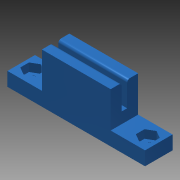
# Autodesk Inventor part: GT2 grip
Saved by Autodesk Inventor 2013 SP2 (Build 170200200, 200)
## iProperties
Created: 2017-01-29
Part Number: GT2 grip
Material: Generic
Document SubType Name: Modeling
Designer: Herman de Vries
Density: 1 g/cm^3
Mass: 5.10381 g
Surface Area: 30.2542 cm^2
Volume: 5.10381 cm^3
Author: Herman de Vries
Autodesk Inventor part; units mm, degrees
ref_plane "YZ Plane" through (0, 0, 0) normal (1, 0, 0) x (0, 1, 0)
ref_plane "XZ Plane" through (0, 0, 0) normal (0, 1, 0) x (-1, 0, 0)
ref_plane "XY Plane" through (0, 0, 0) normal (0, 0, 1) x (1, 0, 0)
sketch "Sketch1" plane through (0, 0, 0) normal (0, 0, 1) x (1, 0, 0)
  line L0 (0, 0) -> (50, 0)
  line L1 (50, 0) -> (50, 10)
  line L2 (50, 10) -> (0, 10)
  line L3 (0, 10) -> (0, 0)
  circle A0 centre (4, 5) radius 1.5
  circle A1 centre (46, 5) radius 1.5
  point P0 (0, 5)
  dimension "d0" = 50
  dimension "d1" = 10
  dimension "d22" = 3
  dimension "d23" = 3
  dimension "d24" = 4
  dimension "d25" = 4
  constraints: 8 end point, 2 centre point, 2 horizontal alignment, 2 parallel, 1 horizontal, 1 midpoint, 1 perpendicular
  measures "d0" distance of L2.end L1.end
  measures "d1" distance of L1.end L0.end
  measures "d22" diameter of A0
  measures "d23" diameter of A1
  measures "d24" distance from line of L3 A0.centre
  measures "d25" distance from line of L1 A1.centre
extrude "Extrusion1" add sketch "Sketch1" along normal blind 5
sketch "Sketch2" plane through (0, 0, 5) normal (0, 0, 1) x (1, 0, 0)
  line L0 (50, 10) -> (0, 10) projected
  line L1 (0, 0) -> (50, 0) projected
  line L2 (12.5, 10) -> (37.5, 10)
  line L3 (37.5, 10) -> (37.5, 6)
  line L4 (37.5, 6) -> (12.5, 6)
  line L5 (12.5, 6) -> (12.5, 10)
  line L6 (12.5, 0) -> (37.5, 0)
  line L7 (37.5, 0) -> (37.5, 4)
  line L8 (37.5, 4) -> (12.5, 4)
  line L9 (12.5, 4) -> (12.5, 0)
  point P0 (25, 10)
  point P1 (25, 10)
  point P2 (25, 0)
  point P3 (25, 0)
  dimension "d14" = 25
  dimension "d15" = 25
  dimension "d31" = 2
  dimension "d32" = 4
  dimension "d33" = 4
  constraints: 16 end point, 4 midpoint, 4 parallel, 2 coincident, 2 horizontal, 2 perpendicular, 2 point on line
  measures "d14" distance of L2.start L2.end
  measures "d15" distance between parallel lines of L9 L7
  measures "d31" distance between parallel lines of L8 L4
  measures "d32" distance of L2.end L3.end
  measures "d33" distance of L6.end L7.end
extrude "Extrusion2" add sketch "Sketch2" along normal blind 13
fillet "Fillet1" radius 1 2 edges at (25, 6, 18) (25, 4, 18)
sketch "Sketch3" plane through (0, 0, 5) normal (0, 0, 1) x (1, 0, 0)
  circle A0 centre (4, 5) radius 1.5 projected
  circle A1 centre (46, 5) radius 1.5 projected
  line L0 (6.75, 6.5877) -> (6.75, 3.4123)
  line L1 (6.75, 3.4123) -> (4, 1.8246)
  line L2 (4, 1.8246) -> (1.25, 3.4123)
  line L3 (1.25, 3.4123) -> (1.25, 6.5877)
  line L4 (1.25, 6.5877) -> (4, 8.1754)
  line L5 (4, 8.1754) -> (6.75, 6.5877)
  line L6 (43.25, 6.5877) -> (46, 8.1754)
  line L7 (46, 8.1754) -> (48.75, 6.5877)
  line L8 (48.75, 6.5877) -> (48.75, 3.4123)
  line L9 (48.75, 3.4123) -> (46, 1.8246)
  line L10 (46, 1.8246) -> (43.25, 3.4123)
  line L11 (43.25, 3.4123) -> (43.25, 6.5877)
  point P0 (0, 0)
  dimension "d39" = 5.5
  dimension "d40" = 5.5
  constraints: 24 end point, 2 coincident, 2 vertical, 26 other
  measures "d39" distance between parallel lines of L0 L3
  measures "d40" distance between parallel lines of L8 L11
extrude "Extrusion3" cut sketch "Sketch3" against normal blind 3
sketch "Sketch4" plane through (0, 0, 5) normal (0, 0, 1) x (1, 0, 0)
  line L0 (12.5, 6) -> (12.5, 10) projected
  line L1 (37.5, 4) -> (37.5, 0) projected
  line L2 (12.5, 6) -> (37.5, 6)
  line L3 (37.5, 6) -> (37.5, 4)
  line L4 (37.5, 4) -> (12.5, 4)
  line L5 (12.5, 4) -> (12.5, 6)
  point P0 (0, 0)
  constraints: 8 end point, 2 parallel, 1 horizontal, 1 perpendicular
extrude "Extrusion4" add sketch "Sketch4" along normal blind 4
equation "\"d15\" = d14"
equation "\"d32\" = d33"
equation "\"d40\" = d39"
body "Solid1"
